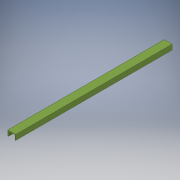
# Autodesk Inventor part: lift rails
Saved by Autodesk Inventor 2017 SP1 (Build 210196100, 196)
## iProperties
Created: 2018-01-12
Part Number: lift rails
Material: Generic
Document SubType Name: Modeling
Designer: Ben
Density: 1 g/cm^3
Appearance: Olive Green
Author: Ben
Autodesk Inventor part; units mm, degrees
ref_plane "YZ Plane" through (0, 0, 0) normal (1, 0, 0) x (0, 1, 0)
ref_plane "XZ Plane" through (0, 0, 0) normal (0, 1, 0) x (-1, 0, 0)
ref_plane "XY Plane" through (0, 0, 0) normal (0, 0, 1) x (1, 0, 0)
sketch "Sketch1" plane through (0, 0, 0) normal (0, 0, 1) x (1, 0, 0)
  line L0 (-16.179, -22.225) -> (-16.179, 0)
  line L1 (-16.179, 0) -> (15.571, 0)
  line L2 (15.571, 0) -> (15.571, -22.225)
  line L3 (15.571, -22.225) -> (18.746, -22.225)
  line L4 (18.746, -22.225) -> (18.746, 3.175)
  line L5 (18.746, 3.175) -> (-19.354, 3.175)
  line L6 (-19.354, 3.175) -> (-19.354, -22.225)
  line L7 (-19.354, -22.225) -> (-16.179, -22.225)
  line L8 (15.571, 0) -> (18.746, 0) construction
  line L9 (-16.179, 0) -> (-19.354, 0) construction
  line L10 (0, 0) -> (0, 3.175) construction
  dimension "d0" = 3.175
  dimension "d1" = 31.75
  dimension "d2" = 25.4
  dimension "d3" = 38.1
  constraints: 22 end point, 8 perpendicular, 5 point on line, 2 equal length, 1 parallel, 1 vertical
  measures "d0" distance of L10.start L10.end
  measures "d1" distance of L0.end L1.end
  measures "d2" distance of L3.end L4.end
  measures "d3" distance of L4.end L5.end
extrude "Extrusion1" add sketch "Sketch1" along normal mid plane 762
body "Solid1"
